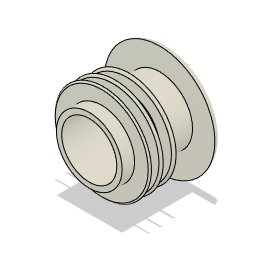
0.885.3303 - Bouchon d'extrémité - IGTE 21482_227061 (Autodesk Fusion 360 design; units mm, degrees)
Autodesk Fusion 360 part; units mm, degrees
sketch "Sketch1" plane through (0, 0, 0) normal (0, 0, 1) x (1, 0, 0)
  circle A0 centre (0, 0) radius 23.5
  dimension "d1" = 47
  constraint coincident A0.centre origin
  measures "d1" diameter of A0
extrude "Extrude1" add sketch "Sketch1" along normal blind 3 makes body 1
fillet "Fillet1" radius 3 1 edges at (-21.9097, -8.498, 0) on bodies 1
sketch "Sketch2" plane through (0, 0, 3) normal (0, 0, 1) x (1, 0, 0)
  circle A0 centre (0, 0) radius 23.5
  circle A1 centre (0, 0) radius 14
  dimension "d5" = 28
  constraint coincident A0.centre A1.centre
  measures "d5" diameter of A1
extrude "Extrude2" add sketch "Sketch2" along normal blind 13 contours A1 bodies 1
sketch "Sketch3" plane through (0, 0, 16) normal (0, 0, 1) x (1, 0, 0)
  circle A0 centre (0, 0) radius 14
  circle A1 centre (0, 0) radius 20
  dimension "d8" = 40
  constraint coincident A0.centre A1.centre
  measures "d8" diameter of A1
extrude "Extrude3" add sketch "Sketch3" along normal blind 1 separate body makes body 2
fillet "Fillet2" radius 1 1 edges at (-18.6465, -7.2323, 17) on bodies 2
sketch "Sketch4" plane through (0, 0, 16) normal (0, 0, 1) x (1, 0, 0)
  circle A0 centre (0, 0) radius 14
  circle A1 centre (0, 0) radius 20.5
extrude "Extrude4" add sketch "Sketch4" along normal blind 6 contours A0 bodies 1 2
sketch "Sketch5" plane through (0, 0, 22) normal (0, 0, 1) x (1, 0, 0)
  circle A0 centre (0, 0) radius 14
  circle A1 centre (0, 0) radius 20.5
  circle A2 centre (0, 0) radius 18.5
  dimension "d14" = 37
  constraint coincident A0.centre A1.centre
  measures "d14" diameter of A2
extrude "Extrude5" add sketch "Sketch5" along normal blind 0.9 separate body contours A1 | A2 makes body 3
fillet "Fillet3" radius 0.9 1 edges at (-19.1127, -7.4131, 22.9) on bodies 3
extrude "Extrude6" add 1 faces at (3.6071, -3.6485, 22) along direction (0, 0, 1) blind 5 on bodies 1 bodies 1 3
sketch "Sketch6" plane through (0, 0, 27) normal (0, 0, 1) x (1, 0, 0)
  circle A0 centre (0, 0) radius 14
  circle A1 centre (0, 0) radius 20.5
  circle A2 centre (0, 0) radius 17
  dimension "d20" = 34
  constraint coincident A0.centre A1.centre
  measures "d20" diameter of A2
extrude "Extrude7" add sketch "Sketch6" along normal blind 0.7 separate body contours A1 | A2 makes body 4
fillet "Fillet4" radius 0.7 1 edges at (-19.1127, -7.4131, 27.7) on bodies 4
extrude "Extrude8" add 1 faces at (3.6071, -3.6485, 27) along direction (0, 0, 1) blind 6 on bodies 1 bodies 1 4
sketch "Sketch7" plane through (0, 0, 33) normal (0, 0, 1) x (1, 0, 0)
  circle A0 centre (0, 0) radius 14
  circle A1 centre (0, 0) radius 20.5
  circle A2 centre (0, 0) radius 11.75
  dimension "d26" = 23.5
  constraint coincident A0.centre A1.centre
  measures "d26" diameter of A2
extrude "Extrude9" cut sketch "Sketch7" against normal blind 30 contours A2 bodies 1
equation "d24 = 30 mm - 13 mm - 6 mm - 5 mm"
